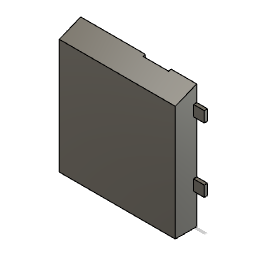
ArduinoCover (Autodesk Fusion 360 design; units mm, degrees)
Autodesk Fusion 360 part; units mm, degrees
sketch "Sketch1" plane through (0, 0, 0) normal (0, 0, 1) x (1, 0, 0) in component "Cover"
  line L0 (20, 20) -> (128, 20)
  line L1 (128, 20) -> (128, 135)
  line L2 (128, 135) -> (20, 135)
  line L3 (20, 135) -> (20, 20)
  dimension "d1" = 20
  dimension "d2" = 20
  dimension "d3" = 115
  dimension "d4" = 108
  constraint horizontal L0
  constraint vertical L1
  constraint horizontal L2
  constraint vertical L3
  measures "d1" horizontal distance of origin L0.start
  measures "d2" vertical distance of origin L0.start
  measures "d3" distance of L0.start L2.end
  measures "d4" distance of L1.end L2.end
extrude "Extrude1" add sketch "Sketch1" along normal blind 20 in component "Cover"
sketch "Sketch2" plane through (0, 0, 0) normal (0, 0, -1) x (-1, 0, 0) in component "Cover"
  line L0 (-20, 20) -> (-20, 135)
  line L1 (-20, 135) -> (-128, 135)
  line L2 (-128, 135) -> (-128, 20)
  line L3 (-128, 20) -> (-20, 20)
  line L4 (-126, 104) -> (-22, 104)
  line L5 (-22, 104) -> (-22, 22)
  line L6 (-22, 22) -> (-126, 22)
  line L7 (-126, 22) -> (-126, 104)
  dimension "d8" = 2
  dimension "d10" = 2
  dimension "d28" = 82
  dimension "d29" = 104
  constraint horizontal L4
  constraint vertical L5
  constraint horizontal L6
  constraint vertical L7
  measures "d8" horizontal distance of L1.end L4.start
  measures "d10" vertical distance of L0.start L5.end
  measures "d28" distance of L4.start L6.end
  measures "d29" distance of L5.end L6.end
extrude "Extrude2" cut sketch "Sketch2" against normal blind 18 contours L4 L5 L6 L7 in component "Cover"
sketch "Sketch3" plane through (20, 0, 0) normal (-1, 0, 0) x (0, 0, 1) in component "Cover"
  line L0 (0, 135) -> (0, 20)
  line L1 (0, 20) -> (20, 20)
  line L2 (20, 20) -> (20, 135)
  line L3 (20, 135) -> (0, 135)
  line L4 (0, 58) -> (14, 58)
  line L5 (14, 58) -> (14, 42)
  line L6 (14, 42) -> (0, 42)
  line L7 (20, 135) -> (0, 135)
  line L8 (0, 135) -> (20, 127)
  line L9 (0, 120) -> (3, 120)
  line L10 (3, 120) -> (3, 110)
  line L11 (3, 110) -> (0, 110)
  line L12 (0, 110) -> (0, 120)
  line L13 (0, 70) -> (3, 70)
  line L14 (3, 70) -> (3, 60)
  line L15 (3, 60) -> (0, 60)
  line L16 (0, 60) -> (0, 70)
  dimension "d13" = 14
  dimension "d14" = 16
  dimension "d16" = 22
  dimension "d30" = 8
  dimension "d51" = 3
  dimension "d52" = 10
  dimension "d53" = 3
  dimension "d54" = 10
  dimension "d55" = 90
  dimension "d56" = 40
  constraint horizontal L4
  constraint vertical L5
  constraint horizontal L6
  constraint coincident L0.start L3.end
  constraint coincident L2.end L3.start
  constraint coincident L0 L4.start
  constraint coincident L0 L6.end
  constraint coincident L2 L8.end
  constraint horizontal L9
  constraint vertical L10
  constraint horizontal L11
  constraint vertical L12
  constraint coincident L0 L9.start
  constraint horizontal L13
  constraint vertical L14
  constraint horizontal L15
  constraint vertical L16
  measures "d13" distance of L5.end L6.end
  measures "d14" distance of L4.end L5.end
  measures "d16" vertical distance of L0.end L6.end
  measures "d30" distance of L2.end L8.end
  measures "d51" distance of L13.start L14
  measures "d52" distance of L13.end L14.end
  measures "d53" distance of L10.end L11.end
  measures "d54" distance of L9.end L10.end
  measures "d55" distance of L0.end L11.end
  measures "d56" distance of L0.end L15.end
sketch "Sketch1 (2)" plane through (0, 20, 0) normal (0, -1, 0) x (1, 0, 0)
  line L0 (20, 0) -> (128, 0)
  line L1 (128, 0) -> (128, 20)
  line L2 (128, 20) -> (20, 20)
  line L3 (20, 20) -> (20, 0)
  line L4 (95, 5) -> (107, 5)
  line L5 (107, 5) -> (107, 10)
  line L6 (107, 10) -> (95, 10)
  line L7 (95, 10) -> (95, 5)
  point P0 (20, 0)
  dimension "d22" = 5
  dimension "d23" = 12
  dimension "d24" = 75
  dimension "d25" = 5
  constraint horizontal L4
  constraint vertical L5
  constraint horizontal L6
  constraint vertical L7
  measures "d22" distance of L4.start L6.end
  measures "d23" distance of L5.end L6.end
  measures "d24" horizontal distance of L4.start P0
  measures "d25" vertical distance of L4.start P0
extrude "Extrude6" cut sketch "Sketch3" against normal up to surface (108 mm away) contours L2 L3 L7 L8 in component "Cover"
sketch "Sketch2 (2)" plane through (0, 0, 0) normal (0, 0, -1) x (-1, 0, 0)
  line L0 (-22, 104) -> (-22, 22)
  line L1 (-22, 22) -> (-126, 22)
  line L2 (-126, 22) -> (-126, 104)
  line L3 (-126, 104) -> (-22, 104)
  line L4 (-20, 20) -> (-20, 135)
  line L5 (-20, 135) -> (-128, 135)
  line L6 (-128, 135) -> (-128, 20)
  line L7 (-128, 20) -> (-20, 20)
  line L8 (-104, 104) -> (-80, 104)
  line L9 (-80, 104) -> (-80, 125)
  line L10 (-80, 125) -> (-104, 125)
  line L11 (-104, 125) -> (-104, 104)
  line L12 (-104, 125) -> (-80, 125)
  line L13 (-80, 125) -> (-80, 135)
  line L14 (-80, 135) -> (-104, 135)
  line L15 (-104, 135) -> (-104, 125)
  dimension "d33" = 21
  dimension "d34" = 24
  dimension "d35" = 22
  dimension "d36" = 24
  constraint horizontal L8
  constraint vertical L9
  constraint horizontal L10
  constraint vertical L11
  constraint coincident L3 L8.start
  constraint horizontal L12
  constraint vertical L13
  constraint horizontal L14
  constraint vertical L15
  constraint coincident L5 L13.end
  measures "d33" distance of L8.end L9.end
  measures "d34" distance of L9.end L10.end
  measures "d35" distance of L2.end L8.start
  measures "d36" distance of L13.end L14.end
extrude "Extrude7" cut sketch "Sketch2 (2)" against normal up to surface (18 mm away) contours L3 L8 L9 L10 L11 L12 in component "Cover"
extrude "Extrude8" cut sketch "Sketch2 (2)" against normal blind 2 contours L5 L10 L12 L13 L14 L15 in component "Cover"
extrude "Extrude9" cut sketch "Sketch3" against normal up to surface (2 mm away) contours L0 L4 L5 L6 in component "Cover"
sketch "Sketch3 (2)" plane through (128, 0, 0) normal (1, 0, 0) x (0, 0, -1)
  line L0 (0, 135) -> (-20, 127)
  line L1 (-20, 127) -> (-20, 20)
  line L2 (-20, 20) -> (0, 20)
  line L3 (0, 20) -> (0, 135)
  line L4 (0, 120) -> (-3, 120)
  line L5 (-3, 120) -> (-3, 110)
  line L6 (-3, 110) -> (0, 110)
  line L7 (0, 110) -> (0, 120)
  line L8 (0, 60) -> (-3, 60)
  line L9 (-3, 60) -> (-3, 50)
  line L10 (-3, 50) -> (0, 50)
  line L11 (0, 50) -> (0, 60)
  dimension "d43" = 3
  dimension "d44" = 10
  dimension "d45" = 10
  dimension "d46" = 3
  dimension "d47" = 30
  dimension "d48" = 50
  constraint horizontal L4
  constraint vertical L5
  constraint horizontal L6
  constraint vertical L7
  constraint coincident L3 L4.start
  constraint horizontal L8
  constraint vertical L9
  constraint horizontal L10
  constraint vertical L11
  constraint coincident L3 L8.start
  measures "d43" distance of L8.start L8.end
  measures "d44" distance of L8.end L9.end
  measures "d45" distance of L4.end L5.end
  measures "d46" distance of L5.end L6.end
  measures "d47" distance of L2.end L10.end
  measures "d48" distance of L6.end L8.start
extrude "Extrude10" add sketch "Sketch3 (2)" along normal blind 10 contours L3 L4 L5 L6 L7 | L3 L8 L9 L10 L11 in component "Cover"
extrude "Extrude11" add sketch "Sketch3" along normal blind 10 contours L0 L9 L10 L11 L12 | L0 L13 L14 L15 L16 in component "Cover"
component "Cover" placed x (1, 0, 0) y (0, 1, 0) z (0, 0, 1) at (0, 0, 0)
